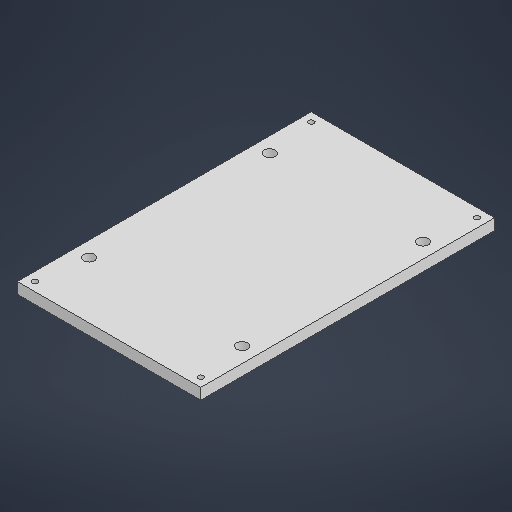
# Autodesk Inventor part: Spincoater Base Mount
Saved by Autodesk Inventor 2025.1 (Build 291241000, 241)
## iProperties
Created: 2025-02-09
Part Number: Spincoater Base Mount
Material: Generic
Document SubType Name: Modeling
Designer: jerem
Density: 1 g/cm^3
Appearance: Default
Author: jerem
Autodesk Inventor part; units mm, degrees
ref_plane "YZ Plane" through (0, 0, 0) normal (1, 0, 0) x (0, 1, 0)
ref_plane "XZ Plane" through (0, 0, 0) normal (0, 1, 0) x (-1, 0, 0)
ref_plane "XY Plane" through (0, 0, 0) normal (0, 0, 1) x (1, 0, 0)
sketch "Sketch1" plane through (0, 0, 0) normal (0, 1, 0) x (-1, 0, 0)
  circle A0 centre (69.3, 81.8) radius 2.5
  circle A1 centre (69.3, -81.8) radius 2.5
  circle A2 centre (-69.3, -81.8) radius 2.5
  circle A3 centre (-69.3, 81.8) radius 2.5
  line L0 (69.3, 81.8) -> (-69.3, 81.8) construction
  line L1 (69.3, 81.8) -> (69.3, -81.8) construction
  line L2 (69.3, -81.8) -> (-69.3, -81.8) construction
  line L3 (0, 0) -> (69.3, 0) construction
  line L4 (-83, -133) -> (83, -133)
  line L5 (83, -133) -> (83, 133)
  line L6 (83, 133) -> (-83, 133)
  line L7 (-83, 133) -> (-83, -133)
  line L8 (-83, -133) -> (83, 133) construction
  line L9 (83, -133) -> (-83, 133) construction
  circle A4 centre (75, 125) radius 2.5
  circle A5 centre (-75, 125) radius 2.5
  circle A6 centre (-75, -125) radius 2.5
  circle A7 centre (75, -125) radius 2.5
  line L10 (75, 125) -> (-75, 125) construction
  line L11 (-75, 125) -> (-75, -125) construction
  line L12 (75, -125) -> (-75, -125) construction
  circle A8 centre (69.3, 81.8) radius 5
  circle A9 centre (-69.3, 81.8) radius 5
  circle A10 centre (-69.3, -81.8) radius 5
  circle A11 centre (69.3, -81.8) radius 5
  point P0 (0, 81.8)
  dimension "d0" = 163.6
  dimension "d1" = 5
  dimension "d2" = 138.6
  dimension "d3" = 69.3
  dimension "d4" = 5
  dimension "d5" = 10
  dimension "d7" = 250
  dimension "d8" = 8
  dimension "d9" = 8
  dimension "d10" = 8
  dimension "d11" = 8
  dimension "d12" = 8
  dimension "d13" = 150
  constraints: 26 end point, 12 centre point, 9 equal radius, 4 coincident, 4 horizontal, 4 midpoint, 4 parallel, 3 perpendicular, 1 vertical
  measures "d0" distance of L0.start L1.end
  measures "d1" diameter of A0
  measures "d2" distance of L0.start L0.end
  measures "d3" distance of L3.start L3.end
  measures "d4" diameter of A4
  measures "d5" diameter of A8
  measures "d7" distance of L10.end L11.end
  measures "d8" distance from line of L10.start L5
  measures "d9" distance from line of L6 L10.start
  measures "d10" distance from line of L4 L12.start
  measures "d11" distance from line of L5 L12.start
  measures "d12" distance from line of L7 L10.end
  measures "d13" distance of L10.start L10.end
extrude "Extrusion1" add sketch "Sketch1" along normal blind 10 contours L7 L6 L5 L4
extrude "Extrusion2" add sketch "Sketch1" along normal blind 3 contours A8 | A9 | A10 | A11
equation "\"d3\" = 0.5 * d2"
equation "\"d9\" = d8"
equation "\"d10\" = d9"
equation "\"d11\" = d8"
equation "\"d12\" = d8"
body "Solid1"
